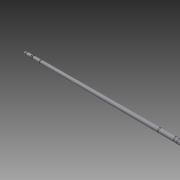
# Autodesk Inventor part: IDLER SHAFT
Saved by Autodesk Inventor 2014 (Build 180170000, 170)
## iProperties
Created: 2013-09-20
Part Number: IDLER SHAFT
Material: Generic
Document SubType Name: Modeling
Designer: Brandon
Density: 1 g/cm^3
Appearance: Default
Author: Brandon
Autodesk Inventor part; units mm, degrees
ref_plane "YZ Plane" through (0, 0, 0) normal (1, 0, 0) x (0, 1, 0)
ref_plane "XZ Plane" through (0, 0, 0) normal (0, 1, 0) x (-1, 0, 0)
ref_plane "XY Plane" through (0, 0, 0) normal (0, 0, 1) x (1, 0, 0)
sketch "Sketch1" plane through (0, 0, 0) normal (0, 1, 0) x (-1, 0, 0)
  line L0 (0, 0) -> (-40, 0) construction
  line L1 (0, 0) -> (0, 0.75)
  line L2 (0, 0.75) -> (-24.16, 0.75)
  line L3 (-24.5, 0.75) -> (-28.5, 0.75)
  line L4 (-28.5, 0.75) -> (-28.84, 0.75) construction
  line L5 (-29.75, 0.75) -> (-32.75, 0.75)
  line L6 (-32.75, 0.75) -> (-33.09, 0.75) construction
  line L7 (-34, 0.75) -> (-34, 0)
  line L8 (-34, 0.75) -> (-33.25, 0.75) construction
  line L9 (-34, 0) -> (0, 0)
  line L10 (-34, 0.6) -> (0, 0.6) construction
  line L11 (-32.75, 0.75) -> (-32.75, 0.6)
  line L12 (-32.75, 0.6) -> (-33.09, 0.6)
  line L13 (-33.09, 0.6) -> (-33.09, 0.75)
  line L14 (-33.09, 0.75) -> (-34, 0.75)
  line L15 (-29.75, 0.75) -> (-29.75, 0.6)
  line L16 (-29.75, 0.6) -> (-29.41, 0.6)
  line L17 (-29.41, 0.6) -> (-29.41, 0.75)
  line L18 (-28.5, 0.75) -> (-28.5, 0.6)
  line L19 (-28.5, 0.6) -> (-28.84, 0.6)
  line L20 (-28.84, 0.6) -> (-28.84, 0.75)
  line L21 (-29.41, 0.75) -> (-29.75, 0.75) construction
  line L22 (-28.84, 0.75) -> (-29.41, 0.75)
  line L23 (-24.5, 0.75) -> (-24.5, 0.6)
  line L24 (-24.5, 0.6) -> (-24.16, 0.6)
  line L25 (-24.16, 0.6) -> (-24.16, 0.75)
  line L26 (-24.16, 0.75) -> (-24.5, 0.75) construction
  line L27 (0, 0) -> (40, 0) construction
  line L28 (0, 0.75) -> (24.16, 0.75)
  line L29 (24.5, 0.75) -> (28.5, 0.75)
  line L30 (28.5, 0.75) -> (28.84, 0.75) construction
  line L31 (29.75, 0.75) -> (32.75, 0.75)
  line L32 (32.75, 0.75) -> (33.09, 0.75) construction
  line L33 (34, 0.75) -> (34, 0)
  line L34 (34, 0.75) -> (33.25, 0.75) construction
  line L35 (34, 0) -> (0, 0)
  line L36 (34, 0.6) -> (0, 0.6) construction
  line L37 (32.75, 0.75) -> (32.75, 0.6)
  line L38 (32.75, 0.6) -> (33.09, 0.6)
  line L39 (33.09, 0.6) -> (33.09, 0.75)
  line L40 (33.09, 0.75) -> (34, 0.75)
  line L41 (29.75, 0.75) -> (29.75, 0.6)
  line L42 (29.75, 0.6) -> (29.41, 0.6)
  line L43 (29.41, 0.6) -> (29.41, 0.75)
  line L44 (28.5, 0.75) -> (28.5, 0.6)
  line L45 (28.5, 0.6) -> (28.84, 0.6)
  line L46 (28.84, 0.6) -> (28.84, 0.75)
  line L47 (29.41, 0.75) -> (29.75, 0.75) construction
  line L48 (28.84, 0.75) -> (29.41, 0.75)
  line L49 (24.5, 0.75) -> (24.5, 0.6)
  line L50 (24.5, 0.6) -> (24.16, 0.6)
  line L51 (24.16, 0.6) -> (24.16, 0.75)
  line L52 (24.16, 0.75) -> (24.5, 0.75) construction
  dimension "d36" = 40
  dimension "d38" = 0.75
  dimension "d39" = 24.5
  dimension "d41" = 4
  dimension "d43" = 1.25
  dimension "d45" = 3
  dimension "d47" = 1.25
  dimension "d50" = 90
  dimension "d51" = 34
  dimension "d52" = 1.2
  dimension "d53" = 0.75
  dimension "d54" = 1.5
  dimension "d55" = 0.34
  dimension "d56" = 0.34
  dimension "d57" = 0.34
  dimension "d58" = 0.34
  constraints: 102 end point, 21 symmetric about line, 14 perpendicular, 11 collinear, 5 vertical, 4 horizontal, 3 point on line, 22 other
  measures "d36" distance of L0.start L0.end
  measures "d38" distance of L0.start L1.end
  measures "d39" distance of L1.end L3.start
  measures "d41" distance of L3.start L3.end
  measures "d43" distance of L3.end L5.start
  measures "d45" distance of L5.start L5.end
  measures "d47" distance of L5.end L7.start
  measures "d50" angle of L7 L8
  measures "d51" distance of L7.end L0.start
  measures "d53" distance between parallel lines of L6 L9
  measures "d54" diameter of L6 L0
  measures "d55" distance of L11.end L12.end
  measures "d56" distance of L15.end L16.end
  measures "d57" distance of L18.end L19.end
  measures "d58" distance of L23.end L24.end
revolve "Revolution2" add sketch "Sketch1" angle 360 about axis through (-34, 0, 0) along (1, 0, 0)
body "Solid2"
